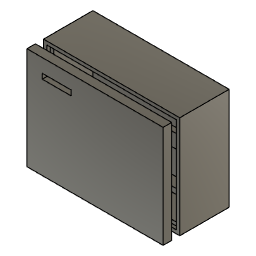
Relay Box (Autodesk Fusion 360 design; units mm, degrees)
Autodesk Fusion 360 part; units mm, degrees
sketch "Skizze1" plane through (0, 0, 0) normal (0, 1, 0) x (1, 0, 0)
  line L0 (0, 0) -> (80, 0)
  line L1 (80, 0) -> (80, 60)
  line L2 (80, 60) -> (0, 60)
  line L3 (0, 60) -> (0, 0)
  line L4 (76, 56) -> (4, 56)
  line L5 (4, 56) -> (4, 4)
  line L6 (4, 4) -> (76, 4)
  line L7 (76, 4) -> (76, 56)
  line L8 (0, 0) -> (80, 0)
  line L9 (80, 0) -> (80, 31)
  line L10 (80, 31) -> (0, 31)
  line L11 (0, 31) -> (0, 0)
  line L12 (0, 60) -> (80, 60)
  line L13 (80, 60) -> (80, 39)
  line L14 (80, 39) -> (0, 39)
  line L15 (0, 39) -> (0, 60)
  dimension "d1" = 80
  dimension "d2" = 60
  dimension "d3" = -4
  dimension "d4" = 80
  dimension "d5" = 31
  dimension "d6" = 80
  dimension "d7" = 21
  constraint horizontal L0
  constraint vertical L1
  constraint horizontal L2
  constraint vertical L3
  constraint coincident L0.start L3.end
  constraint horizontal L8
  constraint vertical L9
  constraint horizontal L10
  constraint vertical L11
  constraint horizontal L12
  constraint vertical L13
  constraint horizontal L14
  constraint vertical L15
  measures "d1" distance of L0.start L0.end
  measures "d2" distance of L0.start L2.end
  measures "d4" distance of L0.start L0.end
  measures "d5" distance of L0.start L10.end
  measures "d6" distance of L2.end L1.end
  measures "d7" distance of L2.end L14.end
extrude "Extrusion1" add sketch "Skizze1" along normal blind 4 makes body 1
extrude "Extrusion2" add sketch "Skizze1" against normal blind 25 contours L0 L1 L3 L5 L6 L7 L8 L9 L10 L11 | L3 L5 L10 L14 | L1 L7 L10 L14 | L1 L2 L3 L4 L5 L7 L12 L13 L14 L15 bodies 1
extrude "Extrusion3" add sketch "Skizze1" against normal blind 3 contours L5 L7 L10 L14 bodies 1
sketch "Skizze2" plane through (0, 0, -60) normal (0, 0, -1) x (1, 0, 0)
  line L0 (0, 25) -> (0, -4)
  line L1 (0, -4) -> (80, -4)
  line L2 (80, -4) -> (80, 25)
  line L3 (80, 25) -> (0, 25)
  line L4 (0, 0) -> (81, 0)
  line L5 (81, 0) -> (81, 6)
  line L6 (81, 6) -> (0, 6)
  line L7 (0, 6) -> (0, 0)
  line L8 (10, 6) -> (70, 6)
  line L9 (70, 6) -> (70, 9)
  line L10 (70, 9) -> (10, 9)
  line L11 (10, 9) -> (10, 6)
  constraint horizontal L4
  constraint vertical L5
  constraint horizontal L6
  constraint vertical L7
  constraint coincident L4.start L7.end
  constraint horizontal L8
  constraint vertical L9
  constraint horizontal L10
  constraint vertical L11
  constraint coincident L6 L8.start
extrude "Extrusion4" cut sketch "Skizze2" against normal blind 5 contours L6 L8 L9 L10 L11 bodies 1
sketch "Skizze3" plane through (0, -25, 0) normal (0, -1, 0) x (1, 0, 0)
  line L0 (76, -4) -> (76, -56)
  line L1 (76, -56) -> (4, -56)
  line L2 (4, -56) -> (4, -4)
  line L3 (4, -4) -> (76, -4)
  line L4 (0, 0) -> (0, -60)
  line L5 (0, -60) -> (80, -60)
  line L6 (80, -60) -> (80, 0)
  line L7 (80, 0) -> (0, 0)
  line L8 (80, -60) -> (0, -60)
  line L9 (0, -60) -> (0, 0)
  line L10 (0, 0) -> (80, 0)
  line L11 (80, 0) -> (80, -60)
  constraint horizontal L8
  constraint vertical L9
  constraint horizontal L10
  constraint vertical L11
  constraint coincident L4.start L7.end
  constraint coincident L5.end L6.start
extrude "Extrusion5" add sketch "Skizze3" along normal blind 5 separate body contours L0 L1 L2 L3 | L4 L5 L6 L7 L8 L9 L10 L11 makes body 2
sketch "Skizze4" plane through (0, -30, 0) normal (0, -1, 0) x (1, 0, 0)
  line L0 (80, 0) -> (0, 0)
  line L1 (0, 0) -> (0, -60)
  line L2 (0, -60) -> (80, -60)
  line L3 (80, -60) -> (80, 0)
  line L4 (80, -60) -> (0, -60)
  line L5 (0, -60) -> (0, -52)
  line L6 (0, -52) -> (80, -52)
  line L7 (80, -52) -> (80, -60)
  line L8 (80, -60) -> (71, -60)
  line L9 (71, -60) -> (71, -35)
  line L10 (71, -35) -> (80, -35)
  line L11 (80, -35) -> (80, -60)
  line L12 (71, -52) -> (54, -52)
  line L13 (54, -52) -> (54, -49)
  line L14 (54, -49) -> (71, -49)
  line L15 (71, -49) -> (71, -52)
  dimension "d18" = 17
  dimension "d19" = 3
  constraint horizontal L4
  constraint vertical L5
  constraint horizontal L6
  constraint vertical L7
  constraint coincident L1 L5.end
  constraint coincident L2.end L3.start
  constraint horizontal L8
  constraint vertical L9
  constraint horizontal L10
  constraint vertical L11
  constraint horizontal L12
  constraint vertical L13
  constraint horizontal L14
  constraint vertical L15
  constraint coincident L6 L12.start
  constraint coincident L9 L12.start
  measures "d18" distance of L12.start L12.end
  measures "d19" distance of L12.start L14.end
extrude "Extrusion6" cut sketch "Skizze4" against normal blind 15 contours L6 L9 L12 L13 L14 L15 bodies 2
sketch "Skizze5" plane through (0, -25, 0) normal (0, 1, 0) x (-1, 0, 0)
  line L0 (-54, -49) -> (-54, -52)
  line L1 (-54, -52) -> (-71, -52)
  line L2 (-71, -52) -> (-71, -49)
  line L3 (-71, -49) -> (-54, -49)
  line L4 (0, 0) -> (-80, 0)
  line L5 (-80, 0) -> (-80, -60)
  line L6 (-80, -60) -> (0, -60)
  line L7 (0, -60) -> (0, 0)
  line L8 (-4, -4) -> (-76, -4)
  line L9 (-76, -4) -> (-76, -56)
  line L10 (-76, -56) -> (-4, -56)
  line L11 (-4, -56) -> (-4, -4)
  line L12 (-2, -2) -> (-78, -2)
  line L13 (-78, -2) -> (-78, -58)
  line L14 (-78, -58) -> (-2, -58)
  line L15 (-2, -58) -> (-2, -2)
  dimension "d22" = -4
  dimension "d23" = -2
extrude "Extrusion7" add sketch "Skizze5" along normal blind 2 contours L12 L13 L14 L15 bodies 2
combine "Kombinieren1" operation cut target body 1 tool bodies 2 keep tools
copy_body "Körper->Berechn1" bodies 1 removing the originals makes body 3 in component "Component"
copy_body "Körper->Berechn2" bodies 2 removing the originals makes body 4 in component "Component'"
move_body "Verschieben1" bodies 4 to x (-1, 0, 0) y (0, 1, 0) z (0, 0, -1) at (80, 0, -60) in component "Component'"
component "Component" placed x (1, 0, 0) y (0, 1, 0) z (0, 0, 1) at (0, 0, 0)
component "Component'" placed x (1, 0, 0) y (0, 1, 0) z (0, 0, 1) at (0, 0, 0)
equation "d22 = 4 mm - 8 mm"
